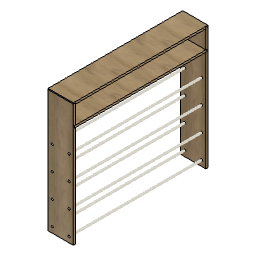
Filament_Rack_Wood_Final (Autodesk Fusion 360 design; units mm, degrees)
Autodesk Fusion 360 part; units mm, degrees
sketch "Sketch11" plane through (0, 0, 0) normal (0, 0, 1) x (1, 0, 0)
  line L0 (0, 0) -> (228.6, 0)
  line L1 (228.6, 0) -> (228.6, -19.05)
  line L2 (228.6, -19.05) -> (0, -19.05)
  line L3 (0, -19.05) -> (0, 0)
  dimension "d134" = 228.6
  dimension "d135" = 19.05
  constraint horizontal L0
  constraint vertical L1
  constraint horizontal L2
  constraint vertical L3
  constraint coincident L0.start L3.end
  measures "d134" distance of L0.start L0.end
  measures "d135" distance of L0.start L2.end
extrude "Extrude5" add sketch "Sketch11" along normal blind 1108.075 makes body 1
sketch "Sketch12" plane through (0, 0, 0) normal (-1, 0, 0) x (0, -1, 0)
  line L0 (0, 0) -> (19.05, 0)
  line L1 (19.05, 0) -> (19.05, 1108.075)
  line L2 (19.05, 1108.075) -> (0, 1108.075)
  line L3 (0, 1108.075) -> (0, 0)
  line L4 (19.05, 1108.075) -> (19.05, 933.45)
  line L5 (19.05, 933.45) -> (9.525, 933.45)
  line L6 (9.525, 933.45) -> (9.525, 914.4)
  line L7 (9.525, 914.4) -> (19.05, 914.4)
  line L8 (19.05, 914.4) -> (19.05, 933.45)
  dimension "d139" = 174.625
  dimension "d140" = 9.525
  dimension "d141" = 19.05
  constraint coincident L1.end L2.start
  constraint perpendicular L2 L4
  constraint horizontal L5
  constraint vertical L6
  constraint horizontal L7
  constraint vertical L8
  measures "d139" distance of L1.end L4.end
  measures "d140" distance of L4.end L5.end
  measures "d141" distance of L4.end L7.end
extrude "Extrude6" cut sketch "Sketch12" against normal blind 228.6 contours L1 L5 L6 L7 L8 bodies 1
sketch "Sketch13" plane through (0, 0, 0) normal (0, 1, 0) x (1, 0, 0)
  line L0 (0, 0) -> (38.1, 0)
  line L1 (38.1, 0) -> (38.1, -50.8)
  line L2 (38.1, -50.8) -> (0, -50.8)
  line L3 (0, -50.8) -> (0, 0)
  circle A0 centre (38.1, -50.8) radius 9.525
  dimension "d145" = 38.1
  dimension "d146" = 50.8
  dimension "d147" = 19.05
  constraint horizontal L0
  constraint vertical L1
  constraint horizontal L2
  constraint vertical L3
  constraint coincident L0.start L3.end
  constraint coincident L1.end L2.start
  measures "d145" distance of L0.start L0.end
  measures "d146" distance of L0.start L2.end
  measures "d147" diameter of A0
extrude "Extrude7" cut sketch "Sketch13" against normal blind 19.05 contours L1 L2 A0 | L1 L2 A0 bodies 1
pattern_linear "R-Pattern2" count 4 spacing 215.9 along (0, 0, 1) count 2 spacing 152.4 along (1, 0, 0) of "Extrude7"
copy_body "Body->Comp13" bodies 1 removing the originals makes body 2 in component "Side 2"
sketch "Sketch1" plane through (0, 0, 0) normal (-1, 0, 0) x (0, -1, 0) in component "Top"
  line L0 (19.05, 914.4) -> (9.525, 914.4)
  line L1 (9.525, 914.4) -> (9.525, 933.45)
  line L2 (9.525, 933.45) -> (19.05, 933.45)
  line L3 (19.05, 933.45) -> (19.05, 1108.075)
  line L4 (19.05, 1108.075) -> (0, 1108.075)
  line L5 (0, 1108.075) -> (0, 0)
  line L6 (0, 0) -> (19.05, 0)
  line L7 (19.05, 0) -> (19.05, 914.4)
  line L8 (0, 1108.075) -> (1219.2, 1108.075)
  line L9 (1219.2, 1108.075) -> (1219.2, 1089.025)
  line L10 (1219.2, 1089.025) -> (0, 1089.025)
  line L11 (0, 1089.025) -> (0, 1108.075)
  dimension "d154" = 1219.2
  dimension "d155" = 19.05
  constraint horizontal L8
  constraint vertical L9
  constraint horizontal L10
  constraint vertical L11
  constraint coincident L4.end L5.start
  measures "d154" distance of L4.end L8.end
  measures "d155" distance of L4.end L10.end
extrude "Extrude1" add sketch "Sketch1" against normal blind 228.6 separate body contours L3 L4 L5 L8 L10 L11 | L3 L8 L9 L10 makes body 3 in component "Top"
sketch "Sketch2" plane through (0, 0, 0) normal (-1, 0, 0) x (0, -1, 0) in component "Top"
  line L0 (0, 1089.025) -> (1219.2, 1089.025)
  line L1 (1219.2, 1089.025) -> (1219.2, 1108.075)
  line L2 (1219.2, 1108.075) -> (0, 1108.075)
  line L3 (0, 1108.075) -> (0, 1089.025)
  line L4 (0, 1089.025) -> (19.05, 1089.025)
  line L5 (19.05, 1089.025) -> (19.05, 1079.5)
  line L6 (19.05, 1079.5) -> (0, 1079.5)
  line L7 (0, 1079.5) -> (0, 1089.025)
  dimension "d158" = 19.05
  dimension "d159" = 9.525
  constraint horizontal L4
  constraint vertical L5
  constraint horizontal L6
  constraint vertical L7
  constraint coincident L0.start L3.end
  measures "d158" distance of L0.start L4.end
  measures "d159" distance of L0.start L6.end
sketch "Sketch3" plane through (0, 0, 0) normal (-1, 0, 0) x (0, -1, 0) in component "Top"
  line L0 (0, 1089.025) -> (1219.2, 1089.025)
  line L1 (1219.2, 1089.025) -> (1219.2, 1108.075)
  line L2 (1219.2, 1108.075) -> (0, 1108.075)
  line L3 (0, 1108.075) -> (0, 1089.025)
  line L4 (1219.2, 1089.025) -> (1200.15, 1089.025)
  line L5 (1200.15, 1089.025) -> (1200.15, 1079.5)
  line L6 (1200.15, 1079.5) -> (1219.2, 1079.5)
  line L7 (1219.2, 1079.5) -> (1219.2, 1089.025)
  dimension "d162" = 19.05
  dimension "d163" = 9.525
  constraint horizontal L4
  constraint vertical L5
  constraint horizontal L6
  constraint vertical L7
  constraint coincident L0.end L1.start
  measures "d162" distance of L0.end L4.end
  measures "d163" distance of L0.end L6.end
sketch "Sketch4" plane through (0, 0, 0) normal (-1, 0, 0) x (0, -1, 0) in component "Top"
  line L0 (0, 1089.025) -> (1219.2, 1089.025)
  line L1 (1219.2, 1089.025) -> (1219.2, 1108.075)
  line L2 (1219.2, 1108.075) -> (0, 1108.075)
  line L3 (0, 1108.075) -> (0, 1089.025)
  line L4 (0, 1089.025) -> (19.05, 1089.025)
  line L5 (19.05, 1089.025) -> (19.05, 1098.55)
  line L6 (19.05, 1098.55) -> (0, 1098.55)
  line L7 (0, 1098.55) -> (0, 1089.025)
  dimension "d166" = 19.05
  dimension "d167" = 9.525
  constraint horizontal L4
  constraint vertical L5
  constraint horizontal L6
  constraint vertical L7
  constraint coincident L0.start L3.end
  measures "d166" distance of L0.start L4.end
  measures "d167" distance of L0.start L6.end
extrude "Extrude4" cut sketch "Sketch4" against normal blind 228.6 contours L0 L3 L4 L5 L6 L7 bodies 3 in component "Top"
pattern_linear "R-Pattern1" count 2 spacing 1200.15 along (0, -1, 0) of "Extrude4" in component "Top"
sketch "Sketch1 (2)" plane through (0, 0, 0) normal (0, 1, 0) x (1, 0, 0) in component "Dowels"
  circle A0 centre (38.1, -50.8) radius 9.525
extrude "Extrude1'" add sketch "Sketch1 (2)" against normal blind 1219.2 separate body makes body 4 in component "Dowels"
pattern_linear "R-Pattern1'" count 4 spacing 215.9 along (0, 0, 1) count 2 spacing 152.4 along (1, 0, 0) of "Extrude1'" makes body 5 at (46.8015, -812.8, 262.8258) makes body 6 at (46.8015, -812.8, 478.7258) makes body 7 at (28.5834, -812.8, 698.1011) makes body 8 at (191.8914, -812.8, 41.3772) makes body 9 at (181.9683, -812.8, 262.4648) makes body 10 at (181.9683, -812.8, 478.3648) makes body 11 at (180.9834, -812.8, 698.1011) in component "Dowels"
sketch "Sketch1 (3)" plane through (0, 0, 0) normal (-1, 0, 0) x (0, -1, 0) in component "Shelf"
  line L0 (19.05, 914.4) -> (9.525, 914.4)
  line L1 (9.525, 914.4) -> (9.525, 933.45)
  line L2 (9.525, 933.45) -> (19.05, 933.45)
  line L3 (19.05, 933.45) -> (19.05, 1108.075)
  line L4 (19.05, 1108.075) -> (0, 1108.075)
  line L5 (0, 1108.075) -> (0, 0)
  line L6 (0, 0) -> (19.05, 0)
  line L7 (19.05, 0) -> (19.05, 914.4)
  line L8 (9.525, 933.45) -> (1209.675, 933.45)
  line L9 (1209.675, 933.45) -> (1209.675, 914.4)
  line L10 (1209.675, 914.4) -> (9.525, 914.4)
  line L11 (9.525, 914.4) -> (9.525, 933.45)
  dimension "d180" = 1200.15
  dimension "d181" = 19.05
  constraint horizontal L8
  constraint vertical L9
  constraint horizontal L10
  constraint vertical L11
  constraint coincident L1.end L2.start
  measures "d180" distance of L1.end L8.end
  measures "d181" distance of L1.end L0.end
extrude "Extrude1''" add sketch "Sketch1 (3)" against normal blind 228.6 separate body contours L0 L1 L2 L8 L9 L10 L11 makes body 12 in component "Shelf"
component "Top" placed x (1, 0, 0) y (0, 1, 0) z (0, 0, 1) at (0, 0, 9.525)
component "Side 2" placed x (1, 0, 0) y (0, 1, 0) z (0, 0, 1) at (0, 0, 0)
component "Side 2" placed x (-1, 0, 0) y (0, -1, 0) z (0, 0, 1) at (228.6, -1219.1206, 0)
component "Dowels" placed x (1, 0, 0) y (0, 1, 0) z (0, 0, 1) at (0, 0, 0)
component "Shelf" placed x (1, 0, 0) y (0, 1, 0) z (0, 0, 1) at (0, 0, 0)
equation "Dado_width = 3/4\""
equation "Dado_Depth = 3/8\""
equation "Rabbet_width = 3/4\""
equation "Rabbet_depth = 3/8\""
equation "Rack_Height = 44\""
equation "Plywood_Thickness = 3/4\""
equation "Rack_Width = 9 in"
equation "Rack_Length = 48 in"
equation "Shelf_Length = Rack_Length - ( Dado_Depth * 2 )"
equation "Dowel_Diameter = 3/4\""
equation "Dowel_Length = 48 in"
equation "Dowel_Horizontal_Spacing = 6 in"
equation "Dowel_Vertical_Spacing = 8.5 in"
equation "d134 = Rack_Width"
equation "d135 = Plywood_Thickness"
equation "d136 = Rack_Height - Rabbet_depth"
equation "Shelf_Offset = 6 7/8\""
equation "d139 = Shelf_Offset"
equation "d140 = Dado_Depth"
equation "d141 = Dado_width"
equation "d142 = -Rack_Width"
equation "First_Dowel_Height = 2 in"
equation "d145 = ( Rack_Width - Dowel_Horizontal_Spacing ) / 2"
equation "d146 = First_Dowel_Height"
equation "d148 = -Plywood_Thickness"
equation "d152 = Dowel_Vertical_Spacing * 3"
equation "d153 = Dowel_Horizontal_Spacing"
equation "d154 = Rack_Length"
equation "d155 = Plywood_Thickness"
equation "d156 = -Rack_Width"
equation "d158 = Rabbet_width"
equation "d159 = Rabbet_depth"
equation "d162 = Rabbet_width"
equation "d163 = Rabbet_depth"
equation "d166 = Rabbet_width"
equation "d167 = Rabbet_depth"
equation "d168 = -Rack_Width"
equation "d172 = Rack_Length - Rabbet_width"
equation "d173 = 0\""
equation "d174 = -Rack_Length"
equation "d178 = Dowel_Vertical_Spacing * 3"
equation "d179 = Dowel_Horizontal_Spacing"
equation "d180 = Shelf_Length"
equation "d181 = Plywood_Thickness"
equation "d182 = -Rack_Width"
